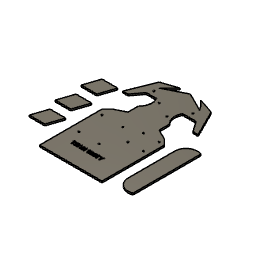
TEAM UNITY 3d (Autodesk Fusion 360 design; units mm, degrees)
Autodesk Fusion 360 part; units mm, degrees
sketch "Sketch1" plane through (0, 0, 0) normal (0, 1, 0) x (1, 0, 0)
  line L0 (60, 0) -> (60, -120)
  line L1 (60, -120) -> (-60, -120)
  line L2 (-60, -120) -> (-60, 0)
  line L3 (30, 40) -> (30, 20)
  line L4 (-30, 20) -> (-30, 40)
  line L5 (-50, 10) -> (-60, 0)
  line L6 (50, 10) -> (60, 0)
  line L7 (-30, 100) -> (-40, 90)
  line L8 (-50, 100) -> (-20, 110)
  line L9 (-20, 110) -> (-30, 100)
  line L10 (30, 100) -> (20, 110)
  line L11 (20, 110) -> (50, 100)
  line L12 (0, 110) -> (-40, 90)
  line L13 (0, 110) -> (35.3846, 92.3077)
  line L14 (-70, 50) -> (-60, 50)
  line L15 (-60, 50) -> (-45, 70)
  line L16 (-50, 100) -> (-70, 50)
  line L17 (50, 100) -> (75, 50)
  line L18 (75, 50) -> (65, 50)
  line L19 (65, 50) -> (51, 70)
  line L20 (35.3846, 92.3077) -> (30, 100)
  line L21 (-45, 70) -> (-25, 70)
  line L22 (25, 70) -> (51, 70)
  arc A0 (-30, 40) -> (-25, 70) centre (-46.4628, 58.1605) ccw
  arc A1 (25, 70) -> (30, 40) centre (46.4628, 58.1605) ccw
  line L23 (-25, 70) -> (-22.1888, 61.5665)
  line L24 (25, 70) -> (22.1888, 61.5665)
  line L25 (-50, 10) -> (-30, 20)
  line L26 (30, 20) -> (50, 10)
  line L27 (110, 0) -> (110, -90)
  line L28 (80, -90) -> (80, 0)
  line L29 (110, 20) -> (110, 0)
  line L30 (110, -110) -> (110, -90)
  arc A2 (80, -90) -> (110, -110) centre (101.6667, -90) ccw
  arc A3 (110, 20) -> (80, 0) centre (101.6667, 0) ccw
  line L31 (-80, 0) -> (-110, 0)
  line L32 (-110, 0) -> (-120, -30)
  line L33 (-120, -30) -> (-90, -30)
  line L34 (-90, -30) -> (-80, 0)
  line L35 (-120, -80) -> (-90, -80)
  line L36 (-90, -80) -> (-80, -50)
  line L37 (-110, -50) -> (-120, -80)
  line L38 (-80, -50) -> (-110, -50)
  line L39 (-120, 20) -> (-90, 20)
  line L40 (-90, 20) -> (-80, 50)
  line L41 (-110, 50) -> (-120, 20)
  line L42 (-80, 50) -> (-110, 50)
  circle A4 centre (-45, 80) radius 1.5
  circle A5 centre (50, 80) radius 1.5
  circle A6 centre (-15, 50) radius 1.5
  circle A7 centre (15, 25) radius 1.5
  circle A8 centre (-50, 0) radius 1.5
  circle A9 centre (-15, 0) radius 1.5
  circle A10 centre (25, 0) radius 1.5
  circle A11 centre (50, 0) radius 1.5
  circle A12 centre (25, -25) radius 1.5
  circle A13 centre (50, -25) radius 1.5
  circle A14 centre (-47.6708, -60) radius 1.5
  circle A15 centre (-5, -60) radius 1.5
  line L43 (-28.9161, -85.8916) -> (-28.8935, -79.245)
  line L44 (-28.8935, -79.245) -> (-31.2672, -79.2369)
  line L45 (-31.2672, -79.2369) -> (-31.2626, -77.8836)
  line L46 (-31.2626, -77.8836) -> (-24.9052, -77.9053)
  line L47 (-24.9052, -77.9053) -> (-24.9099, -79.2586)
  line L48 (-24.9099, -79.2586) -> (-27.2782, -79.2505)
  line L49 (-27.2782, -79.2505) -> (-27.3008, -85.8971)
  line L50 (-27.3008, -85.8971) -> (-28.9161, -85.8916)
  line L51 (-23.8902, -85.9088) -> (-23.863, -77.9088)
  line L52 (-23.863, -77.9088) -> (-17.9312, -77.929)
  line L53 (-17.9312, -77.929) -> (-17.9358, -79.2823)
  line L54 (-17.9358, -79.2823) -> (-22.2523, -79.2676)
  line L55 (-22.2523, -79.2676) -> (-22.2583, -81.0412)
  line L56 (-22.2583, -81.0412) -> (-18.242, -81.0548)
  line L57 (-18.242, -81.0548) -> (-18.2466, -82.4027)
  line L58 (-18.2466, -82.4027) -> (-22.2629, -82.389)
  line L59 (-22.2629, -82.389) -> (-22.2703, -84.5664)
  line L60 (-22.2703, -84.5664) -> (-17.8011, -84.5816)
  line L61 (-17.8011, -84.5816) -> (-17.8057, -85.9295)
  line L62 (-17.8057, -85.9295) -> (-23.8902, -85.9088)
  line L63 (-9.2218, -85.9587) -> (-10.979, -85.9527)
  line L64 (-10.979, -85.9527) -> (-11.6713, -84.1332)
  line L65 (-11.6713, -84.1332) -> (-14.8691, -84.1223)
  line L66 (-14.8691, -84.1223) -> (-15.5355, -85.9372)
  line L67 (-15.5355, -85.9372) -> (-17.249, -85.9314)
  line L68 (-17.249, -85.9314) -> (-14.1059, -77.942)
  line L69 (-14.1059, -77.942) -> (-12.3978, -77.9479)
  line L70 (-12.3978, -77.9479) -> (-9.2218, -85.9587)
  line L71 (-12.1851, -82.7835) -> (-13.2773, -79.8112)
  line L72 (-13.2773, -79.8112) -> (-14.3679, -82.7761)
  line L73 (-14.3679, -82.7761) -> (-12.1851, -82.7835)
  line L74 (-8.3869, -85.9616) -> (-8.3596, -77.9616)
  line L75 (-8.3596, -77.9616) -> (-5.9422, -77.9698)
  line L76 (-5.9422, -77.9698) -> (-4.5092, -83.4318)
  line L77 (-4.5092, -83.4318) -> (-3.0554, -77.9797)
  line L78 (-3.0554, -77.9797) -> (-0.6325, -77.9879)
  line L79 (-0.6325, -77.9879) -> (-0.6598, -85.9879)
  line L80 (-0.6598, -85.9879) -> (-2.1605, -85.9828)
  line L81 (-2.1605, -85.9828) -> (-2.139, -79.6854)
  line L82 (-2.139, -79.6854) -> (-3.7484, -85.9774)
  line L83 (-3.7484, -85.9774) -> (-5.3037, -85.9721)
  line L84 (-5.3037, -85.9721) -> (-6.8648, -79.6693)
  line L85 (-6.8648, -79.6693) -> (-6.8862, -85.9667)
  line L86 (-6.8862, -85.9667) -> (-8.3869, -85.9616)
  line L87 (4.0659, -78.0039) -> (5.6812, -78.0094)
  line L88 (5.6812, -78.0094) -> (5.6665, -82.3423)
  spline S0 degree 2 poles (5.6665, -82.3423) (5.6629, -83.3736) (5.7219, -83.6794) knots 0 0 0 1 1 1
  spline S1 degree 2 poles (5.7219, -83.6794) (5.8239, -84.1709) (6.2131, -84.4697) knots 0 0 0 1 1 1
  spline S2 degree 2 poles (6.2131, -84.4697) (6.6023, -84.7684) (7.2789, -84.7707) knots 0 0 0 1 1 1
  spline S3 degree 2 poles (7.2789, -84.7707) (7.9665, -84.773) (8.3167, -84.4932) knots 0 0 0 1 1 1
  spline S4 degree 2 poles (8.3167, -84.4932) (8.6669, -84.2134) (8.7393, -83.8043) knots 0 0 0 1 1 1
  spline S5 degree 2 poles (8.7393, -83.8043) (8.8116, -83.3953) (8.8148, -82.4458) knots 0 0 0 1 1 1
  line L89 (8.8148, -82.4458) -> (8.8299, -78.0201)
  line L90 (8.8299, -78.0201) -> (10.4452, -78.0256)
  line L91 (10.4452, -78.0256) -> (10.4309, -82.2275)
  spline S6 degree 2 poles (10.4309, -82.2275) (10.4259, -83.6682) (10.293, -84.2625) knots 0 0 0 1 1 1
  spline S7 degree 2 poles (10.293, -84.2625) (10.16, -84.8569) (9.8066, -85.265) knots 0 0 0 1 1 1
  spline S8 degree 2 poles (9.8066, -85.265) (9.4532, -85.6731) (8.863, -85.9139) knots 0 0 0 1 1 1
  spline S9 degree 2 poles (8.863, -85.9139) (8.2729, -86.1547) (7.3233, -86.1515) knots 0 0 0 1 1 1
  spline S10 degree 2 poles (7.3233, -86.1515) (6.1774, -86.1476) (5.5862, -85.8809) knots 0 0 0 1 1 1
  spline S11 degree 2 poles (5.5862, -85.8809) (4.995, -85.6142) (4.6527, -85.1901) knots 0 0 0 1 1 1
  spline S12 degree 2 poles (4.6527, -85.1901) (4.3103, -84.766) (4.2027, -84.3018) knots 0 0 0 1 1 1
  spline S13 degree 2 poles (4.2027, -84.3018) (4.0468, -83.6137) (4.0514, -82.2713) knots 0 0 0 1 1 1
  line L92 (4.0514, -82.2713) -> (4.0659, -78.0039)
  line L93 (12.1369, -86.0315) -> (12.1641, -78.0315)
  line L94 (12.1641, -78.0315) -> (13.7357, -78.0369)
  line L95 (13.7357, -78.0369) -> (16.9917, -83.3904)
  line L96 (16.9917, -83.3904) -> (17.0099, -78.048)
  line L97 (17.0099, -78.048) -> (18.5106, -78.0531)
  line L98 (18.5106, -78.0531) -> (18.4834, -86.0531)
  line L99 (18.4834, -86.0531) -> (16.8626, -86.0475)
  line L100 (16.8626, -86.0475) -> (13.6553, -80.8197)
  line L101 (13.6553, -80.8197) -> (13.6375, -86.0366)
  line L102 (13.6375, -86.0366) -> (12.1369, -86.0315)
  line L103 (20.1423, -86.0587) -> (20.1695, -78.0588)
  line L104 (20.1695, -78.0588) -> (21.7848, -78.0643)
  line L105 (21.7848, -78.0643) -> (21.7576, -86.0642)
  line L106 (21.7576, -86.0642) -> (20.1423, -86.0587)
  line L107 (25.0972, -86.0756) -> (25.1199, -79.429)
  line L108 (25.1199, -79.429) -> (22.7461, -79.4209)
  line L109 (22.7461, -79.4209) -> (22.7507, -78.0676)
  line L110 (22.7507, -78.0676) -> (29.1081, -78.0892)
  line L111 (29.1081, -78.0892) -> (29.1035, -79.4425)
  line L112 (29.1035, -79.4425) -> (26.7351, -79.4345)
  line L113 (26.7351, -79.4345) -> (26.7125, -86.0811)
  line L114 (26.7125, -86.0811) -> (25.0972, -86.0756)
  line L115 (32.2241, -86.0999) -> (32.2355, -82.7329)
  line L116 (32.2355, -82.7329) -> (29.3209, -78.0899)
  line L117 (29.3209, -78.0899) -> (31.2145, -78.0964)
  line L118 (31.2145, -78.0964) -> (33.0864, -81.2678)
  line L119 (33.0864, -81.2678) -> (34.9416, -78.1091)
  line L120 (34.9416, -78.1091) -> (36.8025, -78.1154)
  line L121 (36.8025, -78.1154) -> (33.8453, -82.7493)
  line L122 (33.8453, -82.7493) -> (33.8339, -86.1053)
  line L123 (33.8339, -86.1053) -> (32.2241, -86.0999)
  dimension "d2" = 3
  dimension "d3" = 3
  dimension "d4" = 3
  dimension "d5" = 3
  dimension "d6" = 3
  dimension "d7" = 3
  dimension "d8" = 3
  dimension "d9" = 3
  dimension "d10" = 3
  dimension "d11" = 3
  dimension "d12" = 3
  dimension "d13" = 3
  constraint vertical L0
  constraint horizontal L1
  constraint vertical L2
  constraint vertical L3
  constraint vertical L4
  constraint perpendicular L5 L6
  constraint horizontal L21
  constraint parallel L7 L9
  constraint perpendicular L9 L10
  constraint perpendicular L4 L14
  constraint coincident L13.end L19
  constraint collinear L19 L20
  constraint coincident L22.start L21
  constraint collinear L21 L22
  constraint coincident A0 L23.end
  constraint coincident A1 L24.end
  constraint vertical L27
  constraint vertical L28
  constraint tangent L28 A2
  constraint tangent L28 A3
  constraint horizontal L31
  constraint parallel L31 L33
  constraint parallel L32 L34
  constraint horizontal L38
  constraint parallel L35 L38
  constraint parallel L36 L37
  constraint horizontal L42
  constraint parallel L39 L42
  constraint parallel L40 L41
  measures "d2" diameter of A4
  measures "d3" diameter of A5
  measures "d4" diameter of A6
  measures "d5" diameter of A7
  measures "d6" diameter of A8
  measures "d7" diameter of A9
  measures "d8" diameter of A10
  measures "d9" diameter of A11
  measures "d10" diameter of A12
  measures "d11" diameter of A13
  measures "d12" diameter of A14
  measures "d13" diameter of A15
extrude "Extrude1" add sketch "Sketch1" along normal blind 3 contours L0 L1 L2 L3 L4 L5 L6 L7 L8 L9 L10 L11 L12 L13 L14 L15 L16 L17 L18 L19 L20 L21 L22 A0 A1 L25 L26 | A1 L24 | A0 L23 | L27 L28 L29 L30 A2 A3 | L31 L32 L33 L34 | L35 L36 L37 L38 | L39 L40 L41 L42 | A4 | A5 | A6 | A7 | A8 | A9 | A10 | A11 | A12 | A13 | A14 | A15 | L43 L44 L45 L46 L47 L48 L49 L50 | L51 L52 L53 L54 L55 L56 L57 L58 L59 L60 L61 L62 | L63 L64 L65 L66 L67 L68 L69 L70 | L71 L72 L73 | L74 L75 L76 L77 L78 L79 L80 L81 L82 L83 L84 L85 L86 | L87 L88 S0 S1 S2 S3 S4 S5 L89 L90 L91 S6 S7 S8 S9 S10 S11 S12 S13 L92 | L93 L94 L95 L96 L97 L98 L99 L100 L101 L102 | L103 L104 L105 L106 | L107 L108 L109 L110 L111 L112 L113 L114 | L115 L116 L117 L118 L119 L120 L121 L122 L123 makes body 1 at (-106.6667, 0, 20) makes body 2 at (-106.6667, 0, 70) makes body 3 at (100, 0, 30) makes body 4 at (-20, 0, 40) makes body 5 at (-106.6667, 0, -30)
sketch "Sketch2" plane through (0, 3, 0) normal (0, 1, 0) x (-1, 0, 0)
  line L0 (-25, -70) -> (-51, -70)
  line L1 (-51, -70) -> (-65, -50)
  line L2 (-65, -50) -> (-75, -50)
  line L3 (-75, -50) -> (-50, -100)
  line L4 (-50, -100) -> (-20, -110)
  line L5 (-20, -110) -> (-30, -100)
  line L6 (-30, -100) -> (-35.3846, -92.3077)
  line L7 (-35.3846, -92.3077) -> (0, -110)
  line L8 (0, -110) -> (40, -90)
  line L9 (40, -90) -> (20, -110)
  line L10 (20, -110) -> (50, -100)
  line L11 (50, -100) -> (70, -50)
  line L12 (70, -50) -> (60, -50)
  line L13 (60, -50) -> (45, -70)
  line L14 (45, -70) -> (25, -70)
  line L15 (25, -70) -> (22.1888, -61.5665)
  arc A0 (30, -40) -> (22.1888, -61.5665) centre (46.4628, -58.1605) ccw
  line L16 (30, -40) -> (30, -20)
  line L17 (30, -20) -> (50, -10)
  line L18 (50, -10) -> (60, 0)
  line L19 (60, 0) -> (60, 120)
  line L20 (60, 120) -> (-60, 120)
  line L21 (-60, 120) -> (-60, 0)
  line L22 (-60, 0) -> (-50, -10)
  line L23 (-50, -10) -> (-30, -20)
  line L24 (-30, -20) -> (-30, -40)
  arc A1 (-22.1888, -61.5665) -> (-30, -40) centre (-46.4628, -58.1605) ccw
  line L25 (-22.1888, -61.5665) -> (-25, -70)
  line L26 (34.8282, 92.5775) -> (-33.6731, 93.2874) construction
  line L27 (-33.6731, 93.2874) -> (-33.8097, 80.1143) construction
  line L28 (-33.8097, 80.1143) -> (34.6917, 79.4044) construction
  line L29 (34.6917, 79.4044) -> (34.8282, 92.5775) construction
  dimension "d16" = 7
  text T0 "TEAM UNITY" font "Arial" height 7 bold align left top in box 68.505 x 13.1738 at (34.8282, 92.5775) x (-0.999946, 0.010363) y (-0.010363, -0.999946) spacing 1
extrude "Extrude2" cut sketch "Sketch2" against normal blind 3 text T0 bodies 4 makes body 6 at (-18.6541, 1, 82.0696)
sketch "Sketch3" plane through (0, 3, 0) normal (0, 1, 0) x (-1, 0, 0)
  line L0 (-25, -70) -> (-51, -70)
  line L1 (-51, -70) -> (-65, -50)
  line L2 (-65, -50) -> (-75, -50)
  line L3 (-75, -50) -> (-50, -100)
  line L4 (-50, -100) -> (-20, -110)
  line L5 (-20, -110) -> (-30, -100)
  line L6 (-30, -100) -> (-35.3846, -92.3077)
  line L7 (-35.3846, -92.3077) -> (0, -110)
  line L8 (0, -110) -> (40, -90)
  line L9 (40, -90) -> (20, -110)
  line L10 (20, -110) -> (50, -100)
  line L11 (50, -100) -> (70, -50)
  line L12 (70, -50) -> (60, -50)
  line L13 (60, -50) -> (45, -70)
  line L14 (45, -70) -> (25, -70)
  line L15 (25, -70) -> (22.1888, -61.5665)
  arc A0 (30, -40) -> (22.1888, -61.5665) centre (46.4628, -58.1605) ccw
  line L16 (30, -40) -> (30, -20)
  line L17 (30, -20) -> (50, -10)
  line L18 (50, -10) -> (60, 0)
  line L19 (60, 0) -> (60, 120)
  line L20 (60, 120) -> (-60, 120)
  line L21 (-60, 120) -> (-60, 0)
  line L22 (-60, 0) -> (-50, -10)
  line L23 (-50, -10) -> (-30, -20)
  line L24 (-30, -20) -> (-30, -40)
  arc A1 (-22.1888, -61.5665) -> (-30, -40) centre (-46.4628, -58.1605) ccw
  line L25 (-22.1888, -61.5665) -> (-25, -70)
  line L26 (31.2137, 80.6247) -> (31.2739, 86.4402)
  line L27 (31.2739, 86.4402) -> (32.6872, 86.4255)
  line L28 (32.6872, 86.4255) -> (32.627, 80.61)
  line L29 (32.627, 80.61) -> (34.7039, 80.5885)
  line L30 (34.7039, 80.5885) -> (34.6917, 79.4044)
  line L31 (34.6917, 79.4044) -> (29.1292, 79.462)
  line L32 (29.1292, 79.462) -> (29.1415, 80.6461)
  line L33 (29.1415, 80.6461) -> (31.2137, 80.6247)
  line L34 (19.6802, 79.5599) -> (18.1857, 79.5754)
  line L35 (18.1857, 79.5754) -> (15.4556, 86.6041)
  line L36 (15.4556, 86.6041) -> (16.993, 86.5882)
  line L37 (16.993, 86.5882) -> (17.5877, 84.9919)
  line L38 (17.5877, 84.9919) -> (20.3856, 84.9629)
  line L39 (20.3856, 84.9629) -> (20.9798, 86.5468)
  line L40 (20.9798, 86.5468) -> (22.479, 86.5313)
  line L41 (22.479, 86.5313) -> (19.6802, 79.5599)
  line L42 (-22.2468, 84.0581) -> (-22.2164, 86.9945)
  line L43 (-22.2164, 86.9945) -> (-20.8078, 86.9799)
  line L44 (-20.8078, 86.9799) -> (-20.8384, 84.0339)
  line L45 (-20.8384, 84.0339) -> (-18.3164, 79.9537)
  line L46 (-18.3164, 79.9537) -> (-19.9732, 79.9709)
  line L47 (-19.9732, 79.9709) -> (-21.5918, 82.7572)
  line L48 (-21.5918, 82.7572) -> (-23.2343, 80.0047)
  line L49 (-23.2343, 80.0047) -> (-24.8624, 80.0215)
  line L50 (-24.8624, 80.0215) -> (-22.2468, 84.0581)
  line L51 (-4.5927, 82.2468) -> (-4.5454, 86.8114)
  line L52 (-4.5454, 86.8114) -> (-3.2324, 86.7978)
  line L53 (-3.2324, 86.7978) -> (-3.3049, 79.7981)
  line L54 (-3.3049, 79.7981) -> (-4.68, 79.8124)
  line L55 (-4.68, 79.8124) -> (-7.4964, 84.5165)
  line L56 (-7.4964, 84.5165) -> (-7.5448, 79.8421)
  line L57 (-7.5448, 79.8421) -> (-8.8578, 79.8557)
  line L58 (-8.8578, 79.8557) -> (-8.7853, 86.8553)
  line L59 (-8.7853, 86.8553) -> (-7.3672, 86.8406)
  line L60 (-7.3672, 86.8406) -> (-4.5927, 82.2468)
  line L61 (-16.0457, 81.1144) -> (-15.9855, 86.9299)
  line L62 (-15.9855, 86.9299) -> (-14.5722, 86.9153)
  line L63 (-14.5722, 86.9153) -> (-14.6324, 81.0998)
  line L64 (-14.6324, 81.0998) -> (-12.5555, 81.0782)
  line L65 (-12.5555, 81.0782) -> (-12.5677, 79.8941)
  line L66 (-12.5677, 79.8941) -> (-18.1302, 79.9518)
  line L67 (-18.1302, 79.9518) -> (-18.1179, 81.1359)
  line L68 (-18.1179, 81.1359) -> (-16.0457, 81.1144)
  line L69 (-11.7226, 79.8854) -> (-11.6501, 86.885)
  line L70 (-11.6501, 86.885) -> (-10.2368, 86.8704)
  line L71 (-10.2368, 86.8704) -> (-10.3093, 79.8707)
  line L72 (-10.3093, 79.8707) -> (-11.7226, 79.8854)
  spline S0 degree 3 poles (3.6993, 85.2361) (3.7368, 84.9879) (3.826, 84.399) (3.8218, 83.8032) (3.8193, 83.4585) knots 0 0 0 0 0.075209 0.178405 0.178405 0.178405 0.178405
  line L73 (3.8193, 83.4585) -> (3.7806, 79.7247)
  line L74 (3.7806, 79.7247) -> (2.3673, 79.7394)
  line L75 (2.3673, 79.7394) -> (2.4066, 83.5304)
  spline S1 degree 3 poles (2.4066, 83.5304) (2.4107, 83.7786) (2.4171, 84.1696) (2.3798, 84.5587) (2.3662, 84.7008) knots 0 0 0 0 0.074381 0.117178 0.117178 0.117178 0.117178
  spline S2 degree 3 poles (2.3662, 84.7008) (2.3273, 84.8371) (2.25, 85.108) (2.0437, 85.2998) (1.9413, 85.3952) knots 0 0 0 0 0.041663 0.082805 0.082805 0.082805 0.082805
  spline S3 degree 3 poles (1.9413, 85.3952) (1.8105, 85.4723) (1.5243, 85.641) (1.1914, 85.6566) (1.0105, 85.6651) knots 0 0 0 0 0.044874 0.098214 0.098214 0.098214 0.098214
  spline S4 degree 3 poles (1.0105, 85.6651) (0.83, 85.6623) (0.506, 85.6573) (0.2251, 85.4988) (0.1008, 85.4286) knots 0 0 0 0 0.053119 0.095323 0.095323 0.095323 0.095323
  spline S5 degree 3 poles (0.1008, 85.4286) (0.0084, 85.3442) (-0.1725, 85.1789) (-0.24, 84.9436) (-0.2731, 84.8284) knots 0 0 0 0 0.036734 0.071956 0.071956 0.071956 0.071956
  spline S6 degree 3 poles (-0.2731, 84.8284) (-0.2927, 84.67) (-0.3414, 84.2756) (-0.3452, 83.878) (-0.3475, 83.6401) knots 0 0 0 0 0.047857 0.119139 0.119139 0.119139 0.119139
  line L76 (-0.3475, 83.6401) -> (-0.3876, 79.7679)
  line L77 (-0.3876, 79.7679) -> (-1.8009, 79.7826)
  line L78 (-1.8009, 79.7826) -> (-1.7628, 83.459)
  spline S7 degree 3 poles (-1.7628, 83.459) (-1.7597, 83.8183) (-1.7546, 84.4148) (-1.6653, 85.0043) (-1.6298, 85.2388) knots 0 0 0 0 0.107593 0.178663 0.178663 0.178663 0.178663
  spline S8 degree 3 poles (-1.6298, 85.2388) (-1.5835, 85.403) (-1.4938, 85.7214) (-1.2946, 85.9852) (-1.1981, 86.1129) knots 0 0 0 0 0.050679 0.098258 0.098258 0.098258 0.098258
  spline S9 degree 3 poles (-1.1981, 86.1129) (-1.0822, 86.2264) (-0.8398, 86.4637) (-0.5301, 86.6025) (-0.3686, 86.675) knots 0 0 0 0 0.048273 0.100906 0.100906 0.100906 0.100906
  spline S10 degree 3 poles (-0.3686, 86.675) (-0.1712, 86.7347) (0.2678, 86.8677) (0.7272, 86.8714) (0.9801, 86.8735) knots 0 0 0 0 0.061547 0.136938 0.136938 0.136938 0.136938
  spline S11 degree 3 poles (0.9801, 86.8735) (1.2766, 86.8677) (1.7956, 86.8575) (2.2876, 86.6955) (2.4984, 86.6262) knots 0 0 0 0 0.088347 0.154588 0.154588 0.154588 0.154588
  spline S12 degree 3 poles (2.4984, 86.6262) (2.6587, 86.5446) (2.9654, 86.3884) (3.1993, 86.1364) (3.311, 86.0161) knots 0 0 0 0 0.053473 0.102324 0.102324 0.102324 0.102324
  spline S13 degree 3 poles (3.311, 86.0161) (3.4008, 85.8928) (3.5745, 85.6546) (3.6586, 85.3723) (3.6993, 85.2361) knots 0 0 0 0 0.045375 0.087695 0.087695 0.087695 0.087695
  line L79 (13.3549, 81.1153) -> (13.412, 86.6253)
  line L80 (13.412, 86.6253) -> (14.725, 86.6117)
  line L81 (14.725, 86.6117) -> (14.6525, 79.612)
  line L82 (14.6525, 79.612) -> (12.5373, 79.634)
  line L83 (12.5373, 79.634) -> (11.3168, 84.4218)
  line L84 (11.3168, 84.4218) -> (10.0115, 79.6601)
  line L85 (10.0115, 79.6601) -> (7.8916, 79.6821)
  line L86 (7.8916, 79.6821) -> (7.9641, 86.6817)
  line L87 (7.9641, 86.6817) -> (9.2772, 86.6681)
  line L88 (9.2772, 86.6681) -> (9.2201, 81.1582)
  line L89 (9.2201, 81.1582) -> (10.6666, 86.6537)
  line L90 (10.6666, 86.6537) -> (12.0274, 86.6396)
  line L91 (12.0274, 86.6396) -> (13.3549, 81.1153)
  line L92 (22.9538, 85.3469) -> (22.9661, 86.5263)
  line L93 (22.9661, 86.5263) -> (28.2898, 86.4711)
  line L94 (28.2898, 86.4711) -> (28.2172, 79.4715)
  line L95 (28.2172, 79.4715) -> (23.0272, 79.5253)
  line L96 (23.0272, 79.5253) -> (23.0395, 80.7094)
  line L97 (23.0395, 80.7094) -> (26.8162, 80.6702)
  line L98 (26.8162, 80.6702) -> (26.8323, 82.222)
  line L99 (26.8323, 82.222) -> (23.3182, 82.2584)
  line L100 (23.3182, 82.2584) -> (23.3304, 83.4377)
  line L101 (23.3304, 83.4377) -> (26.8445, 83.4013)
  line L102 (26.8445, 83.4013) -> (26.8643, 85.3064)
  line L103 (26.8643, 85.3064) -> (22.9538, 85.3469)
  circle A2 centre (40, -80) radius 1.5
  circle A3 centre (-35, -80) radius 1.5
  circle A4 centre (15, -65) radius 1.5
  circle A5 centre (-15, -50) radius 1.5
  dimension "d19" = 3
  dimension "d20" = 3
  dimension "d21" = 3
  dimension "d22" = 3
  measures "d19" diameter of A2
  measures "d20" diameter of A3
  measures "d21" diameter of A4
  measures "d22" diameter of A5
extrude "Extrude3" cut sketch "Sketch3" against normal blind 3 contours A2 | A3 | A4 | A5 bodies 4
sketch "Sketch4" plane through (0, 3, 0) normal (0, 1, 0) x (-1, 0, 0)
  circle A0 centre (15, -65) radius 1.5
  circle A1 centre (-35, -80) radius 1.5
  circle A2 centre (40, -80) radius 1.5
  circle A3 centre (-15, -50) radius 1.5
  line L0 (-25, -70) -> (-51, -70)
  line L1 (-51, -70) -> (-65, -50)
  line L2 (-65, -50) -> (-75, -50)
  line L3 (-75, -50) -> (-50, -100)
  line L4 (-50, -100) -> (-20, -110)
  line L5 (-20, -110) -> (-30, -100)
  line L6 (-30, -100) -> (-35.3846, -92.3077)
  line L7 (-35.3846, -92.3077) -> (0, -110)
  line L8 (0, -110) -> (40, -90)
  line L9 (40, -90) -> (20, -110)
  line L10 (20, -110) -> (50, -100)
  line L11 (50, -100) -> (70, -50)
  line L12 (70, -50) -> (60, -50)
  line L13 (60, -50) -> (45, -70)
  line L14 (45, -70) -> (25, -70)
  line L15 (25, -70) -> (22.1888, -61.5665)
  arc A4 (30, -40) -> (22.1888, -61.5665) centre (46.4628, -58.1605) ccw
  line L16 (30, -40) -> (30, -20)
  line L17 (30, -20) -> (50, -10)
  line L18 (50, -10) -> (60, 0)
  line L19 (60, 0) -> (60, 120)
  line L20 (60, 120) -> (-60, 120)
  line L21 (-60, 120) -> (-60, 0)
  line L22 (-60, 0) -> (-50, -10)
  line L23 (-50, -10) -> (-30, -20)
  line L24 (-30, -20) -> (-30, -40)
  arc A5 (-22.1888, -61.5665) -> (-30, -40) centre (-46.4628, -58.1605) ccw
  line L25 (-22.1888, -61.5665) -> (-25, -70)
  line L26 (31.2137, 80.6247) -> (31.2739, 86.4402)
  line L27 (31.2739, 86.4402) -> (32.6872, 86.4255)
  line L28 (32.6872, 86.4255) -> (32.627, 80.61)
  line L29 (32.627, 80.61) -> (34.7039, 80.5885)
  line L30 (34.7039, 80.5885) -> (34.6917, 79.4044)
  line L31 (34.6917, 79.4044) -> (29.1292, 79.462)
  line L32 (29.1292, 79.462) -> (29.1415, 80.6461)
  line L33 (29.1415, 80.6461) -> (31.2137, 80.6247)
  line L34 (19.6802, 79.5599) -> (18.1857, 79.5754)
  line L35 (18.1857, 79.5754) -> (15.4556, 86.6041)
  line L36 (15.4556, 86.6041) -> (16.993, 86.5882)
  line L37 (16.993, 86.5882) -> (17.5877, 84.9919)
  line L38 (17.5877, 84.9919) -> (20.3856, 84.9629)
  line L39 (20.3856, 84.9629) -> (20.9798, 86.5468)
  line L40 (20.9798, 86.5468) -> (22.479, 86.5313)
  line L41 (22.479, 86.5313) -> (19.6802, 79.5599)
  line L42 (-22.2468, 84.0581) -> (-22.2164, 86.9945)
  line L43 (-22.2164, 86.9945) -> (-20.8078, 86.9799)
  line L44 (-20.8078, 86.9799) -> (-20.8384, 84.0339)
  line L45 (-20.8384, 84.0339) -> (-18.3164, 79.9537)
  line L46 (-18.3164, 79.9537) -> (-19.9732, 79.9709)
  line L47 (-19.9732, 79.9709) -> (-21.5918, 82.7572)
  line L48 (-21.5918, 82.7572) -> (-23.2343, 80.0047)
  line L49 (-23.2343, 80.0047) -> (-24.8624, 80.0215)
  line L50 (-24.8624, 80.0215) -> (-22.2468, 84.0581)
  line L51 (-4.5927, 82.2468) -> (-4.5454, 86.8114)
  line L52 (-4.5454, 86.8114) -> (-3.2324, 86.7978)
  line L53 (-3.2324, 86.7978) -> (-3.3049, 79.7981)
  line L54 (-3.3049, 79.7981) -> (-4.68, 79.8124)
  line L55 (-4.68, 79.8124) -> (-7.4964, 84.5165)
  line L56 (-7.4964, 84.5165) -> (-7.5448, 79.8421)
  line L57 (-7.5448, 79.8421) -> (-8.8578, 79.8557)
  line L58 (-8.8578, 79.8557) -> (-8.7853, 86.8553)
  line L59 (-8.7853, 86.8553) -> (-7.3672, 86.8406)
  line L60 (-7.3672, 86.8406) -> (-4.5927, 82.2468)
  line L61 (-16.0457, 81.1144) -> (-15.9855, 86.9299)
  line L62 (-15.9855, 86.9299) -> (-14.5722, 86.9153)
  line L63 (-14.5722, 86.9153) -> (-14.6324, 81.0998)
  line L64 (-14.6324, 81.0998) -> (-12.5555, 81.0782)
  line L65 (-12.5555, 81.0782) -> (-12.5677, 79.8941)
  line L66 (-12.5677, 79.8941) -> (-18.1302, 79.9518)
  line L67 (-18.1302, 79.9518) -> (-18.1179, 81.1359)
  line L68 (-18.1179, 81.1359) -> (-16.0457, 81.1144)
  line L69 (-11.7226, 79.8854) -> (-11.6501, 86.885)
  line L70 (-11.6501, 86.885) -> (-10.2368, 86.8704)
  line L71 (-10.2368, 86.8704) -> (-10.3093, 79.8707)
  line L72 (-10.3093, 79.8707) -> (-11.7226, 79.8854)
  spline S0 degree 3 poles (3.6993, 85.2361) (3.7368, 84.9879) (3.826, 84.399) (3.8218, 83.8032) (3.8193, 83.4585) knots 0 0 0 0 0.075209 0.178405 0.178405 0.178405 0.178405
  line L73 (3.8193, 83.4585) -> (3.7806, 79.7247)
  line L74 (3.7806, 79.7247) -> (2.3673, 79.7394)
  line L75 (2.3673, 79.7394) -> (2.4066, 83.5304)
  spline S1 degree 3 poles (2.4066, 83.5304) (2.4107, 83.7786) (2.4171, 84.1696) (2.3798, 84.5587) (2.3662, 84.7008) knots 0 0 0 0 0.074381 0.117178 0.117178 0.117178 0.117178
  spline S2 degree 3 poles (2.3662, 84.7008) (2.3273, 84.8371) (2.25, 85.108) (2.0437, 85.2998) (1.9413, 85.3952) knots 0 0 0 0 0.041663 0.082805 0.082805 0.082805 0.082805
  spline S3 degree 3 poles (1.9413, 85.3952) (1.8105, 85.4723) (1.5243, 85.641) (1.1914, 85.6566) (1.0105, 85.6651) knots 0 0 0 0 0.044874 0.098214 0.098214 0.098214 0.098214
  spline S4 degree 3 poles (1.0105, 85.6651) (0.83, 85.6623) (0.506, 85.6573) (0.2251, 85.4988) (0.1008, 85.4286) knots 0 0 0 0 0.053119 0.095323 0.095323 0.095323 0.095323
  spline S5 degree 3 poles (0.1008, 85.4286) (0.0084, 85.3442) (-0.1725, 85.1789) (-0.24, 84.9436) (-0.2731, 84.8284) knots 0 0 0 0 0.036734 0.071956 0.071956 0.071956 0.071956
  spline S6 degree 3 poles (-0.2731, 84.8284) (-0.2927, 84.67) (-0.3414, 84.2756) (-0.3452, 83.878) (-0.3475, 83.6401) knots 0 0 0 0 0.047857 0.119139 0.119139 0.119139 0.119139
  line L76 (-0.3475, 83.6401) -> (-0.3876, 79.7679)
  line L77 (-0.3876, 79.7679) -> (-1.8009, 79.7826)
  line L78 (-1.8009, 79.7826) -> (-1.7628, 83.459)
  spline S7 degree 3 poles (-1.7628, 83.459) (-1.7597, 83.8183) (-1.7546, 84.4148) (-1.6653, 85.0043) (-1.6298, 85.2388) knots 0 0 0 0 0.107593 0.178663 0.178663 0.178663 0.178663
  spline S8 degree 3 poles (-1.6298, 85.2388) (-1.5835, 85.403) (-1.4938, 85.7214) (-1.2946, 85.9852) (-1.1981, 86.1129) knots 0 0 0 0 0.050679 0.098258 0.098258 0.098258 0.098258
  spline S9 degree 3 poles (-1.1981, 86.1129) (-1.0822, 86.2264) (-0.8398, 86.4637) (-0.5301, 86.6025) (-0.3686, 86.675) knots 0 0 0 0 0.048273 0.100906 0.100906 0.100906 0.100906
  spline S10 degree 3 poles (-0.3686, 86.675) (-0.1712, 86.7347) (0.2678, 86.8677) (0.7272, 86.8714) (0.9801, 86.8735) knots 0 0 0 0 0.061547 0.136938 0.136938 0.136938 0.136938
  spline S11 degree 3 poles (0.9801, 86.8735) (1.2766, 86.8677) (1.7956, 86.8575) (2.2876, 86.6955) (2.4984, 86.6262) knots 0 0 0 0 0.088347 0.154588 0.154588 0.154588 0.154588
  spline S12 degree 3 poles (2.4984, 86.6262) (2.6587, 86.5446) (2.9654, 86.3884) (3.1993, 86.1364) (3.311, 86.0161) knots 0 0 0 0 0.053473 0.102324 0.102324 0.102324 0.102324
  spline S13 degree 3 poles (3.311, 86.0161) (3.4008, 85.8928) (3.5745, 85.6546) (3.6586, 85.3723) (3.6993, 85.2361) knots 0 0 0 0 0.045375 0.087695 0.087695 0.087695 0.087695
  line L79 (13.3549, 81.1153) -> (13.412, 86.6253)
  line L80 (13.412, 86.6253) -> (14.725, 86.6117)
  line L81 (14.725, 86.6117) -> (14.6525, 79.612)
  line L82 (14.6525, 79.612) -> (12.5373, 79.634)
  line L83 (12.5373, 79.634) -> (11.3168, 84.4218)
  line L84 (11.3168, 84.4218) -> (10.0115, 79.6601)
  line L85 (10.0115, 79.6601) -> (7.8916, 79.6821)
  line L86 (7.8916, 79.6821) -> (7.9641, 86.6817)
  line L87 (7.9641, 86.6817) -> (9.2772, 86.6681)
  line L88 (9.2772, 86.6681) -> (9.2201, 81.1582)
  line L89 (9.2201, 81.1582) -> (10.6666, 86.6537)
  line L90 (10.6666, 86.6537) -> (12.0274, 86.6396)
  line L91 (12.0274, 86.6396) -> (13.3549, 81.1153)
  line L92 (22.9538, 85.3469) -> (22.9661, 86.5263)
  line L93 (22.9661, 86.5263) -> (28.2898, 86.4711)
  line L94 (28.2898, 86.4711) -> (28.2172, 79.4715)
  line L95 (28.2172, 79.4715) -> (23.0272, 79.5253)
  line L96 (23.0272, 79.5253) -> (23.0395, 80.7094)
  line L97 (23.0395, 80.7094) -> (26.8162, 80.6702)
  line L98 (26.8162, 80.6702) -> (26.8323, 82.222)
  line L99 (26.8323, 82.222) -> (23.3182, 82.2584)
  line L100 (23.3182, 82.2584) -> (23.3304, 83.4377)
  line L101 (23.3304, 83.4377) -> (26.8445, 83.4013)
  line L102 (26.8445, 83.4013) -> (26.8643, 85.3064)
  line L103 (26.8643, 85.3064) -> (22.9538, 85.3469)
  circle A6 centre (50, 10) radius 1.5
  circle A7 centre (44.5668, 60) radius 1.5
  circle A8 centre (10, 10) radius 1.5
  circle A9 centre (4.9451, 60.2469) radius 1.5
  circle A10 centre (-20, 0) radius 1.5
  circle A11 centre (-50, 0) radius 1.5
  circle A12 centre (-20, 30) radius 1.5
  circle A13 centre (-50, 30) radius 1.5
  dimension "d25" = 3
  dimension "d26" = 3
  dimension "d27" = 3
  dimension "d28" = 3
  dimension "d29" = 3
  dimension "d30" = 3
  dimension "d31" = 3
  dimension "d32" = 3
  measures "d25" diameter of A6
  measures "d26" diameter of A7
  measures "d27" diameter of A8
  measures "d28" diameter of A9
  measures "d29" diameter of A10
  measures "d30" diameter of A11
  measures "d31" diameter of A12
  measures "d32" diameter of A13
extrude "Extrude4" cut sketch "Sketch4" against normal blind 3 draft 5 contours A6 | A7 | A8 | A9 | A10 | A11 | A12 | A13 bodies 4
